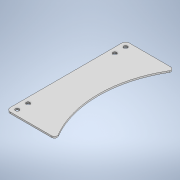
# Autodesk Inventor part: claw_aligner_piece
Saved by Autodesk Inventor 2022 (Build 260153000, 153)
## iProperties
Created: 2021-12-29
Part Number: claw_aligner_piece
Material: Generic
Document SubType Name: Modeling
Designer: Alex
Density: 1 g/cm^3
Appearance: Default
Author: Alex
Autodesk Inventor part; units mm, degrees
ref_plane "YZ Plane" through (0, 0, 0) normal (1, 0, 0) x (0, 1, 0)
ref_plane "XZ Plane" through (0, 0, 0) normal (0, 1, 0) x (-1, 0, 0)
ref_plane "XY Plane" through (0, 0, 0) normal (0, 0, 1) x (1, 0, 0)
sketch "Sketch1" plane through (0, 0, 0) normal (0, 1, 0) x (-1, 0, 0)
  line L0 (-4.445, 0) -> (-38.1, 0)
  line L1 (-38.1, -139.7) -> (-4.445, -139.7)
  line L2 (0, -135.255) -> (0, -4.445)
  arc A0 (-55.8268, -134.9145) -> (-55.8268, -4.7855) centre (-166.37, -69.85) ccw
  line L3 (-38.1, 0) -> (-53.0906, 0)
  line L4 (-53.0906, -139.7) -> (-38.1, -139.7)
  arc A1 (-4.445, -139.7) -> (0, -135.255) centre (-4.445, -135.255) ccw
  arc A2 (0, -4.445) -> (-4.445, 0) centre (-4.445, -4.445) ccw
  arc A3 (-53.0906, 0) -> (-55.8268, -4.7855) centre (-53.0906, -3.175) ccw
  arc A4 (-55.8268, -134.9145) -> (-53.0906, -139.7) centre (-53.0906, -136.525) ccw
  circle A5 centre (-6.35, -6.35) radius 2.2225
  circle A6 centre (-6.35, -19.05) radius 2.2225
  circle A7 centre (-6.35, -133.35) radius 2.2225
  circle A8 centre (-6.35, -120.65) radius 2.2225
  point P0 (0, 0)
  point P1 (0, -139.7)
  point P2 (-58.7867, -139.7)
  point P3 (-58.7867, 0)
  dimension "d0" = 38.1
  dimension "d4" = 4.445
  dimension "d5" = 4.445
  dimension "d6" = 3.175
  dimension "d7" = 4.445
  dimension "d8" = 4.445
  dimension "d9" = 4.445
  dimension "d10" = 4.445
  constraints: 12 point on circle, 10 end point, 9 centre point, 8 tangent, 6 point on line, 2 horizontal, 2 parallel, 1 equal radius
  measures "d0" distance of point (0, -139.7) L1.start
  measures "d4" radius of A1
  measures "d5" radius of A2
  measures "d6" radius of A3
  measures "d7" diameter of A5
  measures "d8" diameter of A6
  measures "d9" diameter of A7
  measures "d10" diameter of A8
extrude "Extrusion1" add sketch "Sketch1" along normal blind 1.778
body "Solid1"
